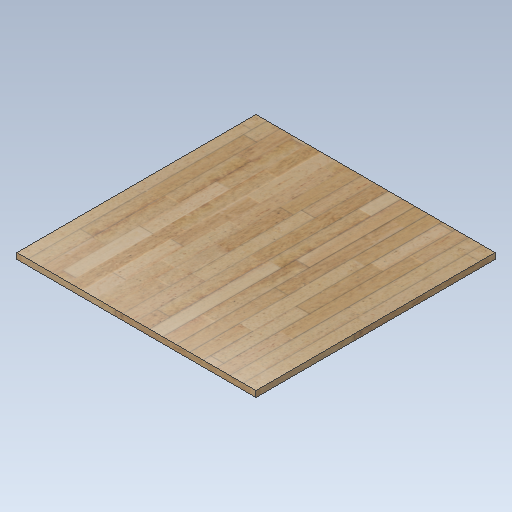
# Autodesk Inventor part: Platform.ver1-1111-2020
Saved by Autodesk Inventor 2020 (Build 240168000, 168)
## iProperties
Created: 2020-01-14
Part Number: Platform.ver1-1111-2020
Material: Wood (Maple)
Document SubType Name: Modeling
Designer: JMHal
Density: 0.67 g/cm^3
Appearance: Natural Maple - Glossy Dark Tint
Author: JMHal
Autodesk Inventor part; units mm, degrees
ref_plane "YZ Plane" through (0, 0, 0) normal (1, 0, 0) x (0, 1, 0)
ref_plane "XZ Plane" through (0, 0, 0) normal (0, 1, 0) x (-1, 0, 0)
ref_plane "XY Plane" through (0, 0, 0) normal (0, 0, 1) x (1, 0, 0)
sketch "Sketch1" plane through (0, 0, 0) normal (0, 1, 0) x (-1, 0, 0)
  line L0 (0, 0) -> (1016, 0)
  line L1 (1016, 0) -> (1016, -1016)
  line L2 (1016, -1016) -> (0, -1016)
  line L3 (0, -1016) -> (0, 0)
  dimension "d0" = 1016
  dimension "d1" = 1016
  constraints: 8 end point, 2 parallel, 1 horizontal, 1 perpendicular
  measures "d0" distance of L1.end L2.end
  measures "d1" distance of L0.end L1.end
extrude "Extrusion1" add sketch "Sketch1" along normal blind 25.4
body "Solid1"
